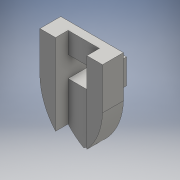
# Autodesk Inventor part: GeneralCraftShape3
Saved by Autodesk Inventor 2016 (Build 200138000, 138)
## iProperties
Created: 2019-01-14
Part Number: GeneralCraftShape3
Material: Generic
Document SubType Name: Modeling
Designer: LinJie
Density: 1 g/cm^3
Appearance: Default
Author: LinJie
Autodesk Inventor part; units mm, degrees
ref_plane "YZ Plane" through (0, 0, 0) normal (1, 0, 0) x (0, 1, 0)
ref_plane "XZ Plane" through (0, 0, 0) normal (0, 1, 0) x (-1, 0, 0)
ref_plane "XY Plane" through (0, 0, 0) normal (0, 0, 1) x (1, 0, 0)
sketch "Sketch3" plane through (0, 0, 0) normal (0, 1, 0) x (-1, 0, 0)
  line L0 (150, 0) -> (-150, 0)
  line L1 (-150, 0) -> (-150, 300)
  line L2 (-150, 300) -> (150, 300)
  line L3 (150, 300) -> (150, 0)
  circle A0 centre (0, 0) radius 150
  arc A1 (0, -150) -> (150, 100) centre (-149.8365, 109.9019) ccw
  arc A2 (-150, 100) -> (0, -150) centre (149.8365, 109.9019) ccw
  dimension "d6" = 300
  dimension "d7" = 300
  dimension "d8" = 100
  dimension "d9" = 100
  dimension "d10" = 300
  dimension "d11" = 300
  constraints: 8 end point, 6 point on circle, 3 centre point, 2 coincident, 2 parallel, 2 point on line, 1 horizontal, 1 midpoint, 1 perpendicular, 1 vertical alignment
  measures "d6" distance between parallel lines of L3 L1
  measures "d7" distance between parallel lines of L2 L0
  measures "d8" distance of L0.end A2.start
  measures "d9" distance of L0.start A1.end
  measures "d10" radius of A1
  measures "d11" radius of A2
extrude "Extrusion2" add sketch "Sketch3" along normal blind 100 contours A1 A2 L0 | L0 A2 A0 A1 | A1 A0 A2 L1 L2 L3
sketch "Sketch4" plane through (-150, 0, 300) normal (0, 0, 1) x (1, 0, 0)
  line L0 (75, 0) -> (225, 0)
  line L1 (225, 0) -> (225, 60)
  line L2 (225, 60) -> (75, 60)
  line L3 (75, 60) -> (75, 0)
  line L4 (0, 0) -> (300, 0) projected
  point P0 (150, 0)
  point P1 (150, 0)
  dimension "d14" = 60
  dimension "d15" = 150
  constraints: 8 end point, 2 midpoint, 2 parallel, 1 horizontal, 1 perpendicular
  measures "d14" distance between parallel lines of L0 L2
  measures "d15" distance between parallel lines of L3 L1
extrude "Extrusion3" cut sketch "Sketch4" against normal through all
sketch "Sketch5" plane through (-75, 60, 300) normal (0, -1, 0) x (1, 0, 0)
  line L0 (0, -388.7146) -> (0, 0) projected
  line L1 (150, 0) -> (150, -388.7146) projected
  line L2 (0, -100) -> (150, -100)
  line L3 (150, -100) -> (150, -200)
  line L4 (150, -200) -> (0, -200)
  line L5 (0, -200) -> (0, -100)
  point P0 (75, -300)
  dimension "d18" = 100
  dimension "d19" = 100
  constraints: 8 end point, 2 parallel, 2 point on line, 1 horizontal, 1 perpendicular
  measures "d18" distance between parallel lines of L4 L2
  measures "d19" distance from line of L1.start L2
extrude "Extrusion4" cut sketch "Sketch5" against normal through all
sketch "Sketch6" plane through (0, 100, 0) normal (0, 1, 0) x (1, 0, 0)
  line L0 (-75, -200) -> (-75, -100) projected
  line L1 (-75, -100) -> (75, -100) projected
  line L2 (75, -100) -> (75, -200) projected
  line L3 (75, -200) -> (-75, -200) projected
  line L4 (-150, -100) -> (-150, -300) projected
  line L5 (-150, -300) -> (150, -300) projected
  line L6 (150, -300) -> (150, -100) projected
  arc A0 (150, -100) -> (0, 150) centre (-149.8365, -109.9019) ccw projected
  arc A1 (0, 150) -> (-150, -100) centre (149.8365, -109.9019) ccw projected
  line L7 (85, -90) -> (-85, -90)
  line L8 (-85, -90) -> (-85, -210)
  line L9 (-85, -210) -> (85, -210)
  line L10 (85, -210) -> (85, -90)
  point P0 (0, 0)
  dimension "d22" = 10
  constraints: 8 end point, 3 other
  measures "d22" distance between parallel lines of L1 L7
extrude "Extrusion5" add sketch "Sketch6" along normal blind 80 contours L10 L9 L8 L7
sketch "Sketch7" plane through (0, 100, 0) normal (0, 1, 0) x (1, 0, 0)
  line L0 (85, -90) -> (-85, -90) construction
  line L1 (50, -90) -> (-50, -90)
  line L2 (-50, -90) -> (-50, 0)
  line L3 (-50, 0) -> (50, 0)
  line L4 (50, 0) -> (50, -90)
  point P0 (0, 0)
  point P1 (0, -90)
  point P2 (0, 0)
  dimension "d25" = 100
  constraints: 8 end point, 3 midpoint, 2 parallel, 1 coincident, 1 horizontal, 1 perpendicular, 1 point on line
  measures "d25" distance between parallel lines of L2 L4
extrude "Extrusion6" add sketch "Sketch7" along normal blind 60
body "Solid2"
